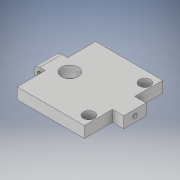
# Autodesk Inventor part: ABI_Deckel
Saved by Autodesk Inventor 2018 (Build 220112000, 112)
## iProperties
Created: 2019-11-22
Part Number: ABI_Deckel
Material: Generisch
Document SubType Name: Modeling
Designer: Dubsky
Density: 1 g/cm^3
Appearance: Vorgabe
Author: Dubsky
Autodesk Inventor part; units mm, degrees
ref_plane "YZ Plane" through (0, 0, 0) normal (1, 0, 0) x (0, 1, 0)
ref_plane "XZ Plane" through (0, 0, 0) normal (0, 1, 0) x (-1, 0, 0)
ref_plane "XY Plane" through (0, 0, 0) normal (0, 0, 1) x (1, 0, 0)
sketch "Skizze1" plane through (0, 0, 0) normal (0, 0, 1) x (1, 0, 0)
  line L0 (-40, -35) -> (40, -35)
  line L1 (40, -35) -> (40, 35)
  line L2 (40, 35) -> (-40, 35)
  line L3 (-40, 35) -> (-40, -35)
  line L4 (-40, -35) -> (40, 35) construction
  line L5 (40, -35) -> (-40, 35) construction
  point P0 (0, 0)
  dimension "d0" = 80
  dimension "d1" = 70
  constraints: 12 end point, 2 midpoint, 2 parallel, 1 horizontal, 1 perpendicular
  measures "d0" distance between parallel lines of L1 L3
  measures "d1" distance between parallel lines of L0 L2
extrude "Extrusion1" add sketch "Skizze1" along normal blind 10
sketch "Skizze2" plane through (0, 0, 10) normal (0, 0, 1) x (1, 0, 0)
  line L0 (-40, 35) -> (-30, 35)
  line L1 (-30, 35) -> (-30, 10)
  line L2 (-30, 10) -> (-40, 10)
  line L3 (-40, 10) -> (-40, 35)
  line L4 (-40, 35) -> (-40, -35) projected
  line L5 (-30, -35) -> (-40, -35)
  line L6 (-40, -35) -> (-40, -10)
  line L7 (-40, -10) -> (-30, -10)
  line L8 (-30, -10) -> (-30, -35)
  line L9 (40, 35) -> (-40, 35) projected
  line L10 (40, -35) -> (40, 35) projected
  line L11 (30, 35) -> (40, 35)
  line L12 (40, 35) -> (40, 10)
  line L13 (40, 10) -> (30, 10)
  line L14 (30, 10) -> (30, 35)
  line L15 (30, -10) -> (40, -10)
  line L16 (40, -10) -> (40, -35)
  line L17 (40, -35) -> (30, -35)
  line L18 (30, -35) -> (30, -10)
  point P0 (0, 0)
  dimension "d4" = 10
  dimension "d5" = 10
  dimension "d6" = 20
  dimension "d7" = 20
  dimension "d8" = 25
  dimension "d9" = 25
  constraints: 32 end point, 8 parallel, 5 point on line, 4 horizontal, 4 perpendicular
  measures "d4" distance between parallel lines of L4 L1
  measures "d5" distance between parallel lines of L14 L12
  measures "d6" distance between parallel lines of L7 L2
  measures "d7" distance between parallel lines of L15 L13
  measures "d8" distance between parallel lines of L9 L13
  measures "d9" distance between parallel lines of L9 L2
extrude "Extrusion2" cut sketch "Skizze2" against normal blind 10
sketch "Skizze3" plane through (0, 0, 10) normal (0, 0, 1) x (1, 0, 0)
  line L0 (-30, -35) -> (30, -35) projected
  line L1 (-30, 10) -> (-40, 10) projected
  line L2 (40, -10) -> (40, 10) projected
  line L3 (30, -35) -> (30, -10) projected
  point P0 (0, 0)
  point P1 (24, 25)
  point P2 (24, -25)
  dimension "d12" = 10
  dimension "d13" = 50
  dimension "d17" = 16
  measures "d12" distance from line of L0 point (24, -25)
  measures "d13" distance of point (24, -25) point (24, 25)
  measures "d17" distance from line of L2 point (24, -25)
hole "Bohrung1" at (24, 25, 10) at (24, -25, 10) direction (0, 0, -1) diameter 10 end through all
sketch "Skizze4" plane through (0, 0, 10) normal (0, 0, 1) x (1, 0, 0)
  line L0 (40, -10) -> (40, 10) projected
  line L1 (-30, 10) -> (-40, 10) projected
  point P0 (0, 0)
  point P1 (-18, 0)
  dimension "d25" = 58
  dimension "d26" = 10
  measures "d25" distance from line of L0 point (-18, 0)
  measures "d26" distance from line of L1 point (-18, 0)
hole "Bohrung2" at (-18, 0, 10) direction (0, 0, -1) diameter 15 end through all
sketch "Skizze5" plane through (-40, -10, 10) normal (0, -1, 0) x (1, 0, 0)
  line L0 (0, 0) -> (10, 0) projected
  line L1 (10, 0) -> (10, -10) projected
  point P0 (40, -10)
  point P1 (5, -5)
  dimension "d34" = 5
  dimension "d35" = 5
  measures "d34" distance from line of L0 point (5, -5)
  measures "d35" distance from line of L1 point (5, -5)
hole "Bohrung3" at (-35, -10, 5) direction (0, 1, 0) diameter 4 end through all
sketch "Skizze6" plane through (40, -10, 0) normal (1, 0, 0) x (0, 0, -1)
  line L0 (0, 20) -> (-10, 20) projected
  line L1 (0, 0) -> (0, 20) projected
  point P0 (0, 10)
  point P1 (-5, 10)
  dimension "d43" = 10
  dimension "d44" = 5
  measures "d43" distance from line of L0 point (-5, 10)
  measures "d44" distance from line of L1 point (-5, 10)
hole "Bohrung4" at (40, 0, 5) direction (-1, 0, 0) diameter 4 depth 10 tip angle 118
fillet "Rundung1" radius 5 2 edges at (-40, 0, 0) (-40, 0, 10)
